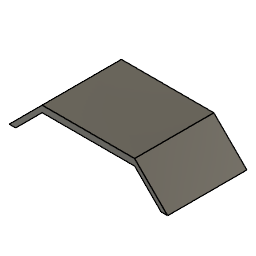
bottom bent plate (~recovered) (Autodesk Fusion 360 design; units mm, degrees)
part number: 2026-08-05-14-44-23-786
Autodesk Fusion 360 part; units mm, degrees
sketch "Sketch1" plane through (0, 0, 0) normal (0, 0, 1) x (1, 0, 0)
  line L0 (44.45, 38.1) -> (-44.45, 38.1)
  line L1 (-44.45, 38.1) -> (-44.45, -38.1)
  line L2 (-44.45, -38.1) -> (44.45, -38.1)
  line L3 (44.45, -38.1) -> (44.45, 38.1)
  line L4 (44.45, 38.1) -> (-44.45, -38.1) construction
  line L5 (-44.45, 38.1) -> (44.45, -38.1) construction
  dimension "d1" = 88.9
  dimension "d2" = 76.2
  constraint horizontal L0
  constraint perpendicular L0 L1
  constraint parallel L0 L2
  constraint parallel L1 L3
  constraint coincident L4 origin
  constraint coincident L5 origin
  measures "d1" distance of L1.end L2.end
  measures "d2" distance of L0.end L1.end
extrude "Extrude1" add sketch "Sketch1" along normal blind 6.35
sketch "Sketch2" plane through (0, 0, 0) normal (0, 1, 0) x (1, 0, 0)
  line L0 (44.45, -6.35) -> (76.2, 25.4)
  line L1 (44.45, 0) -> (69.85, 25.4)
  line L2 (69.85, 25.4) -> (76.2, 25.4)
  line L3 (0, -50.8) -> (0, 63.5)
  line L4 (-69.85, 25.4) -> (-76.2, 25.4)
  line L5 (-44.45, 0) -> (-69.85, 25.4)
  line L6 (-44.45, -6.35) -> (-76.2, 25.4)
  line L7 (-44.45, -6.35) -> (-44.45, 0)
  line L8 (44.45, -6.35) -> (44.45, 0)
  constraint parallel L0 L1
  constraint horizontal L2
  constraint vertical L3
  constraint symmetric L0.start L3 L6.start
  constraint symmetric L0.end L3 L4.end
  constraint symmetric L1.start L3 L5.start
  constraint symmetric L1.end L3 L4.start
  constraint vertical L7
extrude "Extrude2" add sketch "Sketch2" along normal blind 38.1 and the other way blind 38.1
